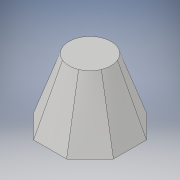
# Autodesk Inventor part: 練習一
Saved by Autodesk Inventor 2017 (Build 210142000, 142)
## iProperties
Part Number: 練習一
Material: 一般
Document SubType Name: Modeling
Designer: user
Density: 1 g/cm^3
Appearance: 預設
Author: user
Autodesk Inventor part; units mm, degrees
ref_plane "YZ Plane" through (0, 0, 0) normal (1, 0, 0) x (0, 1, 0)
ref_plane "XY Plane" through (0, 0, 0) normal (0, 0, 1) x (1, 0, 0)
sketch "草圖1" plane through (0, 0, 0) normal (0, 1, 0) x (-1, 0, 0)
  circle A0 centre (0, 0) radius 10
  dimension "d0" = 20
  constraints: 1 centre point, 1 coincident
  measures "d0" diameter of A0
ref_plane "工作平面1" through (0, -30, 0) normal (0, 1, 0) x (-1, 0, 0)
sketch "草圖2" plane through (0, -30, 0) normal (0, 1, 0) x (-1, 0, 0)
  line L0 (7.8701, -19) -> (-7.8701, -19)
  line L1 (-7.8701, -19) -> (-19, -7.8701)
  line L2 (-19, -7.8701) -> (-19, 7.8701)
  line L3 (-19, 7.8701) -> (-7.8701, 19)
  line L4 (-7.8701, 19) -> (7.8701, 19)
  line L5 (7.8701, 19) -> (19, 7.8701)
  line L6 (19, 7.8701) -> (19, -7.8701)
  line L7 (19, -7.8701) -> (7.8701, -19)
  line L8 (0, 0) -> (0, -16.976)
  dimension "d2" = 38
  constraints: 18 end point, 1 coincident, 1 parallel, 1 vertical, 17 other
  measures "d2" distance between parallel lines of L7 L3
loft "斷面混成1" add profiles "草圖1", "草圖2"
